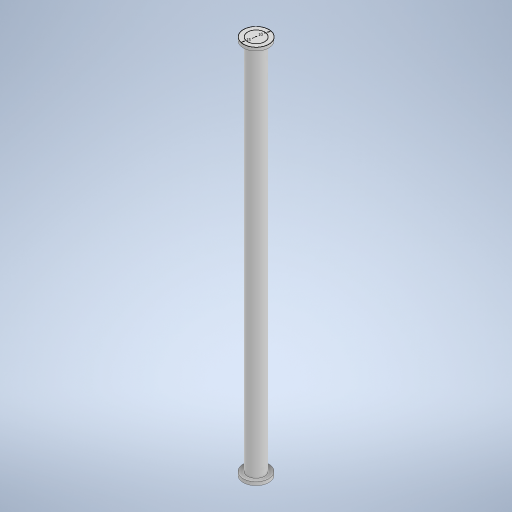
# Autodesk Inventor part: Part2
Saved by Autodesk Inventor 2023.2 (Build 272271000, 271)
## iProperties
Created: 2025-04-10
Part Number: Part2
Material: Generic
Document SubType Name: Modeling
Designer: MEKTROBOT
Density: 1 g/cm^3
Appearance: Default
Author: MEKTROBOT
Autodesk Inventor part; units mm, degrees
ref_plane "YZ Plane" through (0, 0, 0) normal (1, 0, 0) x (0, 1, 0)
ref_plane "XZ Plane" through (0, 0, 0) normal (0, 1, 0) x (-1, 0, 0)
ref_plane "XY Plane" through (0, 0, 0) normal (0, 0, 1) x (1, 0, 0)
sketch "Sketch1" plane through (0, 0, 0) normal (0, 1, 0) x (-1, 0, 0)
  circle A0 centre (0, 0) radius 5
  circle A1 centre (0, 0) radius 7.5
  dimension "d0" = 10
  dimension "d1" = 15
  constraints: 2 centre point, 2 coincident
  measures "d0" diameter of A0
  measures "d1" diameter of A1
extrude "Extrusion1" add sketch "Sketch1" against normal blind 2
extrude "Extrusion2" add sketch "Sketch1" against normal blind 112 contours A0
mirror "Mirror1" about plane through (0, -112, 0) normal (0, -1, 0) of "Extrusion2", "Extrusion1"
body "Solid1"
